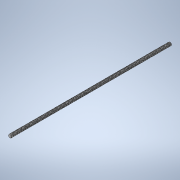
# Autodesk Inventor part: Lead Screw D8-P2 (ACME)
Saved by Autodesk Inventor 2020 (Build 240168000, 168)
## iProperties
Created: 2019-10-21
Part Number: Lead Screw D8-P2 (ACME)
Material: Generic
Document SubType Name: Modeling
Designer: Johnson Ebenezer R
Density: 1 g/cm^3
Appearance: Default
Author: Johnson Ebenezer R
## iProperties of the stored document _3DPrint.ipt
Created: 2019-10-21
Part Number: _3DPrint
Material: Generic
Document SubType Name: Modeling
Designer: Johnson Ebenezer R
Density: 1 g/cm^3
Appearance: Default
Author: Johnson Ebenezer R
Autodesk Inventor part; units mm, degrees
ref_plane "YZ Plane" through (0, 0, 0) normal (1, 0, 0) x (0, 1, 0)
ref_plane "XZ Plane" through (0, 0, 0) normal (0, 1, 0) x (-1, 0, 0)
ref_plane "XY Plane" through (0, 0, 0) normal (0, 0, 1) x (1, 0, 0)
sketch "Sketch1" plane through (0, 0, 0) normal (0, 0, 1) x (1, 0, 0)
  circle A0 centre (0, 0) radius 4
  dimension "d0" = 8
  constraints: 1 centre point, 1 coincident
  measures "d0" diameter of A0
extrude "D8 Rod (400mm)" add sketch "Sketch1" along normal blind 400
chamfer "Chamfer1" distance 1 angle 45 2 edges at (-4, 0, 0) (-4, 0, 400)
sketch "Sketch2" plane through (0, 0, 0) normal (0, 1, 0) x (-1, 0, 0)
  line L0 (4, 0.6293) -> (3, 0.3707) construction
  line L1 (0, 0) -> (0, -1.2586) construction
  line L2 (4, 0) -> (-4, 0) projected
  line L3 (4, 0) -> (4, -1.2586) construction
  line L4 (3, 0) -> (3, -1.2586) construction
  line L5 (4, -0.3707) -> (3, -0.6293)
  line L6 (3, -0.6293) -> (3, -1.3707)
  line L7 (3, -1.3707) -> (4, -1.6293)
  line L8 (4, 0.3707) -> (4, -0.3707) construction
  line L9 (4, -0.3707) -> (4, -1.6293)
  dimension "p" = 2
  dimension "d17" = 29
  dimension "d18" = 1
  dimension "d19" = 0.7414
  constraints: 18 end point, 6 point on line, 5 vertical, 2 horizontal alignment, 2 midpoint, 1 equal length
  measures "p" distance of L7.end L8.start
  measures "d17" angle of L7 L5
  measures "d18" distance between parallel lines of L3 L4
  measures "d19" distance of L6.end L5.end
coil "P2 ACME Thread" sketch "Sketch2" operation cut axis through (0, 0, 0) along (0, 0, 1) pitch 2 turns 261 hand right
equation "\"d18\" = 0.5 * p"
equation "\"d19\" = 0.3707 * p"
body "Solid1"
